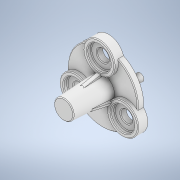
# Autodesk Inventor part: tamiya-slim-tire-hub
Saved by Autodesk Inventor 2021 (Build 250183000, 183)
## iProperties
Created: 2023-10-14
Part Number: tamiya-slim-tire-hub
Material: 一般
Document SubType Name: Modeling
Designer: takag
Density: 1 g/cm^3
Appearance: 滑らか - 白
Author: takag
Autodesk Inventor part; units mm, degrees
ref_plane "YZ Plane" through (0, 0, 0) normal (1, 0, 0) x (0, 1, 0)
ref_plane "XZ Plane" through (0, 0, 0) normal (0, 1, 0) x (-1, 0, 0)
ref_plane "XY Plane" through (0, 0, 0) normal (0, 0, 1) x (1, 0, 0)
sketch "スケッチ1" plane through (0, 0, 0) normal (0, 0, 1) x (1, 0, 0)
  circle A0 centre (0, 0) radius 9
  dimension "d0" = 18
  constraints: 1 centre point, 1 coincident
  measures "d0" diameter of A0
extrude "押し出し1" add sketch "スケッチ1" along normal blind 1.5
sketch "スケッチ2" plane through (0, 0, 0) normal (0, 0, 1) x (1, 0, 0)
  circle A0 centre (0, 7) radius 4
  point P0 (0, 0)
  dimension "d3" = 8
  dimension "d4" = 7
  constraints: 1 centre point
  measures "d3" diameter of A0
  measures "d4" distance of point (0, 0) A0.centre
extrude "押し出し2" add sketch "スケッチ2" along normal blind 2.5
pattern_circular "円形状パターン1" count 3 over 360 about axis through (0, 0, 0) along (0, 0, 1) of "押し出し2"
sketch "スケッチ3" plane through (0, 7, 2.5) normal (0, 0, 1) x (1, 0, 0)
  circle A0 centre (0, 0) radius 1.5
  point P0 (0, -7)
  dimension "d10" = 3
  constraints: 1 centre point
  measures "d10" diameter of A0
extrude "押し出し3" cut sketch "スケッチ3" against normal through all
sketch "スケッチ4" plane through (0, 7, 2.5) normal (0, 0, 1) x (1, 0, 0)
  circle A0 centre (0, 0) radius 3
  point P0 (0, -7)
  dimension "d13" = 6
  constraints: 1 centre point
  measures "d13" diameter of A0
extrude "押し出し4" cut sketch "スケッチ4" against normal blind 1
pattern_circular "円形状パターン2" count 3 over 360 about axis through (0, 0, 0) along (0, 0, 1) of "押し出し4", "押し出し3"
sketch "スケッチ5" plane through (0, 0, 1.5) normal (0, 0, 1) x (1, 0, 0)
  circle A0 centre (0, 0) radius 3
  dimension "d19" = 6
  constraints: 1 centre point, 1 coincident
  measures "d19" diameter of A0
sketch "スケッチ6" plane through (0, 0, 0) normal (1, 0, 0) x (0, 1, 0)
  line L0 (8.1429, 1.5) -> (-0.7517, 1.5) projected
  line L1 (0, 1.5) -> (3, 1.5)
  line L2 (0, 1.5) -> (0, 11.5)
  line L3 (0, 11.5) -> (2.5, 11.5)
  line L4 (2.5, 11.5) -> (3, 1.5)
  point P0 (0, 0)
  dimension "d20" = 3
  dimension "d21" = 10
  dimension "d22" = 2.5
  constraints: 8 end point, 2 perpendicular, 2 point on line
  measures "d20" distance of L1.start L1.end
  measures "d21" distance of L1.start L2.end
  measures "d22" distance of L2.end L3.end
revolve "回転1" add sketch "スケッチ6" angle 360 about axis through (0, 0, 1.5) along (0, 0, 1)
sketch "スケッチ7" plane through (0, 0, 0) normal (0, 0, -1) x (-1, 0, 0)
  arc A0 (0, 3) -> (-2.5981, -1.5) centre (0, 0) ccw projected
  line L0 (0, 0) -> (-6.0622, 3.5)
  line L1 (0, 0) -> (7, 0) construction
  circle A1 centre (-6.0622, 3.5) radius 1
  dimension "d24" = 7
  dimension "d25" = 150
  dimension "d26" = 2
  constraints: 4 end point, 1 centre point, 1 coincident, 1 equal length, 1 horizontal
  measures "d24" distance of L0.start L0.end
  measures "d25" angle of L1 L0
  measures "d26" diameter of A1
extrude "押し出し5" add sketch "スケッチ7" along normal blind 2
pattern_circular "円形状パターン3" count 3 over 360 about axis through (0, 0, 0) along (0, 0, 1) of "押し出し5"
sketch "スケッチ8" plane through (0, 0, 0) normal (1, 0, 0) x (0, 1, 0)
  line L0 (11, 2.5) -> (3, 2.5) projected
  line L1 (3, 1.5) -> (3, 2.5) projected
  line L2 (2.5, 11.5) -> (3, 1.5) projected
  line L3 (-2.5, 11.5) -> (2.5, 11.5) projected
  line L4 (2.75, 6.5) -> (3.5, 2.5)
  line L5 (3.5, 2.5) -> (3.6875, 1.5)
  line L6 (3, 1.5) -> (8.1429, 1.5) projected
  line L7 (-1.5, 1.5) -> (3, 1.5) projected
  line L8 (3, 1.5) -> (2.75, 6.5)
  line L9 (2.75, 6.5) -> (2.05, 10.2335)
  line L10 (2.05, 10.2335) -> (2.05, 1.5)
  point P0 (0, 0)
  dimension "d32" = 0.5
  dimension "d33" = 5
  constraints: 10 end point, 4 point on line, 1 collinear, 1 midpoint, 1 perpendicular
  measures "d32" distance from line of L4.end L1
  measures "d33" distance from line of L3 L4.start
extrude "押し出し6" add sketch "スケッチ8" along normal mid plane 1
pattern_circular "円形状パターン4" count 3 over 360 about axis through (0, 0, 6.5) along (0, 0, -1) of "押し出し6"
fillet "フィレット1" radius 0.2 13 edges at (0, -2.5, 11.5) (7.5622, -0.9019, 2.5) (9.5263, -5.5, 2.5) (0, 11, 2.5) (-3, 7, 2.5) (-9.5263, -5.5, 2.5) (-4.5622, -6.0981, 2.5) (-1.5, 7, 1.5) (-3, 7, 1.5) (7.5622, -0.9019, 1.5) (6.8122, -2.201, 1.5) (-4.5622, -6.0981, 1.5) (-5.3122, -4.799, 1.5)
fillet "フィレット2" radius 0.2 3 edges at (7.7942, 4.5, 1.5) (-7.7942, 4.5, 1.5) (0, -9, 1.5)
sketch "スケッチ9" plane through (0, 0, 0) normal (0, 0, -1) x (-1, 0, 0)
  circle A0 centre (0, 0) radius 1.5
  dimension "d41" = 3
  constraints: 1 centre point, 1 coincident
  measures "d41" diameter of A0
extrude "押し出し7" cut sketch "スケッチ9" against normal blind 10
